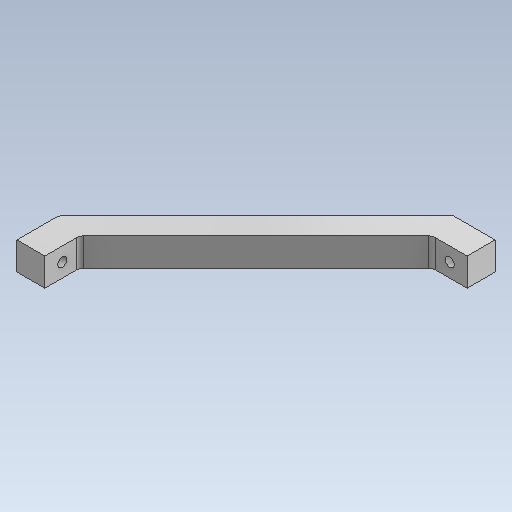
# Autodesk Inventor part: Ranforsare_Imprimanta
Saved by Autodesk Inventor 2020 (Build 240168000, 168)
## iProperties
Created: 2020-12-09
Part Number: Ranforsare_Imprimanta
Material: ABS Plastic
Document SubType Name: Modeling
Designer: Botoca
Mass: 92.9028 g
Surface Area: 201.441 cm^2
Volume: 87.6441 cm^3
Density: 1.06 g/cm^3
Appearance: Smooth - White
Description: Ranforsare
Author: Botoca
Subject: 024
Autodesk Inventor part; units mm, degrees
ref_plane "YZ Plane" through (0, 0, 0) normal (1, 0, 0) x (0, 1, 0)
ref_plane "XZ Plane" through (0, 0, 0) normal (0, 1, 0) x (-1, 0, 0)
ref_plane "XY Plane" through (0, 0, 0) normal (0, 0, 1) x (1, 0, 0)
sketch "Sketch1" plane through (0, 0, 0) normal (0, 0, 1) x (1, 0, 0)
  line L0 (0, 0) -> (0, 30)
  line L1 (0, 30) -> (141.4214, 171.4214)
  line L2 (141.4214, 171.4214) -> (171.4214, 171.4214)
  line L3 (-11.5144, -3.3847) -> (12.7866, -3.3847) construction
  line L4 (171.4214, 171.4214) -> (171.4214, 151.4214)
  line L5 (171.4214, 151.4214) -> (146.4214, 151.4214)
  line L6 (146.4214, 151.4214) -> (20, 25)
  line L7 (20, 25) -> (20, 0)
  line L8 (20, 0) -> (0, 0)
  dimension "d0" = 90
  dimension "d1" = 30
  dimension "d4" = 45
  dimension "d5" = 200
  dimension "d6" = 20
  dimension "d7" = 20
  dimension "d27" = 30
  dimension "d29" = 5
  constraints: 18 end point, 4 perpendicular, 2 coincident, 2 horizontal, 1 parallel, 1 point on line
  measures "d0" angle of L2 L0
  measures "d1" distance of L0.start L0.end
  measures "d4" angle of L0 L1
  measures "d5" distance of L1.end L0.end
  measures "d6" distance of L2.end L4.end
  measures "d7" distance of L7.end L0.start
  measures "d27" distance of L1.end L2.end
  measures "d29" horizontal distance of L5.end point (141.421, 171.421)
extrude "Extrusion1" add sketch "Sketch1" along normal blind 20
sketch "Sketch2" plane through (20, 0, 0) normal (1, 0, 0) x (0, 0, -1)
  line L0 (0, 0) -> (-20, 0) projected
  line L1 (-20, 0) -> (-20, 25) projected
  point P0 (-10, 12.5)
  point P1 (-10, 0)
  point P2 (-20, 12.5)
  constraints: 2 midpoint, 1 horizontal alignment, 1 vertical alignment
sketch "Sketch3" plane through (146.4214, 151.4214, 0) normal (0, -1, 0) x (1, 0, 0)
  line L0 (0, 20) -> (25, 20) projected
  line L1 (25, 0) -> (25, 20) projected
  point P0 (-146.4214, 0)
  point P1 (12.5, 10)
  point P2 (12.5, 20)
  point P3 (25, 10)
  constraints: 2 midpoint, 1 horizontal alignment, 1 vertical alignment
hole "Hole1" at (20, 12.5, 10) direction (-1, 0, 0) diameter 6.5 end through all
hole "Hole2" at (158.9214, 151.4214, 10) direction (0, 1, 0) diameter 6.5 end through all
fillet "Fillet1" radius 5 3 edges at (20, 25, 10) (0, 30, 10) (146.4214, 151.4214, 10)
body "Solid1"
